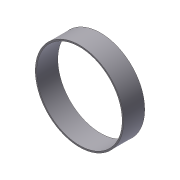
# Autodesk Inventor part: FlyWheel_TreadMount_Jan21
Saved by Autodesk Inventor 2012 (Build 160160000, 160)
## iProperties
Created: 2012-01-22
Part Number: FlyWheel_TreadMount_Jan21
Material: Aluminum-6061
Document SubType Name: Modeling
Designer: JesseK
Mass: 220.499 g
Surface Area: 549.144 cm^2
Volume: 81.3649 cm^3
Density: 2.71 g/cm^3
Author: JesseK
Autodesk Inventor part; units mm, degrees
ref_plane "YZ Plane" through (0, 0, 0) normal (1, 0, 0) x (0, 1, 0)
ref_plane "XZ Plane" through (0, 0, 0) normal (0, 1, 0) x (-1, 0, 0)
ref_plane "XY Plane" through (0, 0, 0) normal (0, 0, 1) x (1, 0, 0)
sketch "Sketch1" plane through (0, 0, 0) normal (0, 0, 1) x (1, 0, 0)
  circle A0 centre (0, 0) radius 90.17
  circle A1 centre (0, 0) radius 93.345
  dimension "d0" = 180.34
  dimension "d1" = 3.175
  constraints: 2 centre point, 2 coincident
  measures "d0" diameter of A0
  measures "d1" radial gap between concentric circles of A0 A1
extrude "Extrusion1" add sketch "Sketch1" along normal blind 44.45
body "Solid1"
